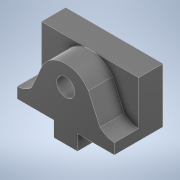
# Autodesk Inventor part: pieza 4. MRKE
Saved by Autodesk Inventor 2021 (Build 250183000, 183)
## iProperties
Created: 2020-10-13
Part Number: pieza 4. MRKE
Material: Steel, Wrought
Document SubType Name: Modeling
Designer: kenii
Density: 7.85 g/cm^3
Appearance: Smooth - Black
Author: kenii
Autodesk Inventor part; units mm, degrees
ref_plane "YZ Plane" through (0, 0, 0) normal (1, 0, 0) x (0, 1, 0)
ref_plane "XZ Plane" through (0, 0, 0) normal (0, 1, 0) x (-1, 0, 0)
ref_plane "XY Plane" through (0, 0, 0) normal (0, 0, 1) x (1, 0, 0)
sketch "Sketch1" plane through (0, 0, 0) normal (0, 0, 1) x (1, 0, 0)
  line L0 (24.25, 0) -> (39.75, 0)
  line L1 (64, 10) -> (64, 46)
  line L2 (64, 46) -> (0, 46)
  line L3 (0, 46) -> (0, 10)
  line L4 (24.25, 0) -> (24.25, 10)
  line L5 (24.25, 10) -> (0, 10)
  line L6 (39.75, 0) -> (39.75, 10)
  line L7 (39.75, 10) -> (64, 10)
  point P0 (0, 0)
  dimension "d0" = 64
  dimension "d2" = 24.25
  dimension "d3" = 10
  constraints: 16 end point, 3 perpendicular, 2 parallel, 2 point on line, 1 horizontal
  measures "d0" distance of L2.end L1.end
  measures "d2" distance of L0.start point (0, 0)
  measures "d3" distance of L0.start L4.end
extrude "Extrusion1" add sketch "Sketch1" along normal blind 16
sketch "Sketch2" plane through (0, 0, 16) normal (0, 0, 1) x (1, 0, 0)
  line L0 (24.25, 10) -> (24.25, 0) projected
  line L1 (24.25, 10) -> (24.25, 0)
  line L2 (24.25, 0) -> (39.75, 0) projected
  line L3 (24.25, 0) -> (39.75, 0)
  line L4 (39.75, 0) -> (39.75, 10) projected
  line L5 (39.75, 0) -> (39.75, 10)
  line L6 (39.75, 10) -> (64, 10) projected
  line L7 (39.75, 10) -> (64, 10)
  line L8 (64, 10) -> (64, 17)
  line L9 (64, 10) -> (64, 46) projected
  line L10 (0, 10) -> (24.25, 10) projected
  line L11 (0, 10) -> (0, 17)
  line L12 (0, 46) -> (0, 10) projected
  arc A0 (0, 17) -> (9.4683, 21.008) centre (-0.759, 31.9808) ccw
  arc A1 (54.5317, 21.008) -> (64, 17) centre (64.759, 31.9808) ccw
  line L13 (17.0879, 38.0812) -> (9.4683, 21.008)
  line L14 (46.9121, 38.0812) -> (54.5317, 21.008)
  arc A2 (46.9121, 38.0812) -> (17.0879, 38.0812) centre (32, 28) ccw
  point P0 (0, 0)
  dimension "d7" = 7
  dimension "d9" = 30
  dimension "d10" = 30
  dimension "d11" = 7
  constraints: 16 end point, 6 point on circle, 3 centre point, 3 collinear, 2 point on line, 1 perpendicular
  measures "d7" distance of L6.end L8.end
  measures "d9" diameter of A0
  measures "d10" diameter of A1
  measures "d11" distance of L10.start L11.end
extrude "Extrusion2" add sketch "Sketch2" along normal blind 16
sketch "Sketch3" plane through (0, 0, 32) normal (0, 0, 1) x (1, 0, 0)
  circle A0 centre (32, 32.647) radius 6
  line L0 (0, 46) -> (0, 17) projected
  line L1 (64, 17) -> (64, 46) projected
  point P0 (0, 0)
  dimension "d14" = 12
  dimension "d15" = 32
  dimension "d16" = 32
  constraints: 1 centre point
  measures "d14" diameter of A0
  measures "d15" distance from line of L0 A0.centre
  measures "d16" distance from line of L1 A0.centre
extrude "Extrusion3" cut sketch "Sketch3" against normal blind 10
sketch "Sketch5" plane through (24.25, 0, 0) normal (0, -1, 0) x (1, 0, 0)
  circle A0 centre (8.0074, 24) radius 4
  circle A1 centre (8.4927, 8) radius 4
  line L0 (0, 32) -> (15.5, 32) projected
  line L1 (0, 0) -> (15.5, 0) projected
  point P0 (-24.25, 0)
  dimension "d22" = 8
  dimension "d23" = 8
  dimension "d26" = 8
  dimension "d27" = 8
  constraints: 2 centre point
  measures "d22" diameter of A0
  measures "d23" diameter of A1
  measures "d26" distance from line of A0.centre L0
  measures "d27" distance from line of L1 A1.centre
extrude "Extrusion5" cut sketch "Sketch5" against normal blind 10
body "Solid1"
